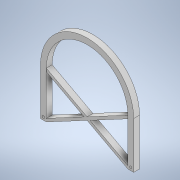
# Autodesk Inventor part: łapka
Saved by Autodesk Inventor 2020 (Build 240168000, 168)
## iProperties
Created: 2023-02-09
Part Number: łapka
Material: Ogólny
Document SubType Name: Modeling
Designer: User
Density: 1 g/cm^3
Appearance: Domyślna
Author: User
Autodesk Inventor part; units mm, degrees
ref_plane "YZ Plane" through (0, 0, 0) normal (1, 0, 0) x (0, 1, 0)
ref_plane "XZ Plane" through (0, 0, 0) normal (0, 1, 0) x (-1, 0, 0)
ref_plane "XY Plane" through (0, 0, 0) normal (0, 0, 1) x (1, 0, 0)
sketch "Szkic1" plane through (0, 0, 0) normal (0, 0, 1) x (1, 0, 0)
  circle A0 centre (0, 0) radius 20
  circle A1 centre (0, 0) radius 17.5
  line L0 (-20, 0) -> (-17.5, 0)
  line L1 (-17.5, 0) -> (-17.5, -20)
  line L2 (-17.5, -20) -> (-20, -20)
  line L3 (-20, -20) -> (-20, 0)
  line L4 (17.5, 0) -> (20, 0)
  line L5 (20, 0) -> (20, -20)
  line L6 (20, -20) -> (17.5, -20)
  line L7 (17.5, -20) -> (17.5, 0)
  circle A2 centre (-18.75, -18.75) radius 0.5
  circle A3 centre (18.75, -18.75) radius 0.5
  line L8 (-20, 0) -> (17.5, -20)
  line L9 (-17.5, 0) -> (20, -20)
  line L10 (-20, -20) -> (17.5, 0)
  line L11 (-17.5, -20) -> (20, 0)
  point P0 (17.5, -18.6667)
  point P1 (1.25, -10)
  point P2 (17.4469, -1.3616)
  point P3 (0, -9.3333)
  point P4 (-17.4469, -1.3616)
  point P5 (-1.25, -10)
  point P6 (-17.5, -18.6667)
  point P7 (0, -10.6667)
  dimension "d1" = 35
  dimension "d0" = 40
  dimension "d2" = 20
  dimension "d3" = 2.5
  dimension "d4" = 2.5
  dimension "d5" = 20
  dimension "d8" = 1
  dimension "d9" = 1.25
  constraints: 24 end point, 4 parallel, 3 centre point, 2 coincident, 2 horizontal, 2 perpendicular, 2 point on circle, 1 point on line, 3 other
  measures "d0" diameter of A0
  measures "d2" distance between parallel lines of L2 L0
  measures "d3" distance of L0.start L0.end
  measures "d4" distance of L4.start L4.end
  measures "d5" distance of L4.end L5.end
  measures "d8" diameter of A2
  measures "d9" distance from line of L2 A2.centre
extrude "Wyciągnięcie proste3" add sketch "Szkic1" along normal blind 2.5 contours L4 A1 L0 A0 | L5 L9 L7 A0 | L11 L7 L4 | A0 L7 L11 | L8 L1 A0 | A0 L1 L10 L3 | L0 L1 L8 | A1 L11 L9 L10 | L6 L7 L9 | L9 L10 L8 A1 | L10 L1 L2 | L9 L7 L8 A0 | A0 L8 A1 L9 | L9 L11 L8 L10 | L10 A1 L11 A0 | A0 L11 L1 L10 | A1 L8 L11 L9 | L8 L11 A1 L10
